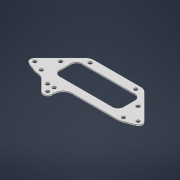
# Autodesk Inventor part: gusset-2-3.25-fulll-brace
Saved by Autodesk Inventor 2021 (Build 250183000, 183)
## iProperties
Created: 2020-11-04
Part Number: gusset-2-3.25-fulll-brace
Material: Generic
Document SubType Name: Modeling
Designer: Carlos Stewart
Density: 1 g/cm^3
Appearance: Default
Author: Carlos Stewart
Autodesk Inventor part; units mm, degrees
ref_plane "YZ Plane" through (0, 0, 0) normal (1, 0, 0) x (0, 1, 0)
ref_plane "XZ Plane" through (0, 0, 0) normal (0, 1, 0) x (-1, 0, 0)
ref_plane "XY Plane" through (0, 0, 0) normal (0, 0, 1) x (1, 0, 0)
sketch "Sketch1" plane through (0, 0, 0) normal (0, 1, 0) x (-1, 0, 0)
  line L0 (-37.8542, 0.1524) -> (35.8058, 0.1524)
  line L1 (43.4258, -7.4676) -> (43.4258, -23.2918)
  line L2 (35.8058, -30.9118) -> (-37.8542, -30.9118)
  line L3 (-45.4742, -23.2918) -> (-45.4742, -7.4676)
  arc A0 (-37.8542, 0.1524) -> (-45.4742, -7.4676) centre (-37.8542, -7.4676) ccw
  arc A1 (-45.4742, -23.2918) -> (-37.8542, -30.9118) centre (-37.8542, -23.2918) ccw
  arc A2 (35.8058, -30.9118) -> (43.4258, -23.2918) centre (35.8058, -23.2918) ccw
  arc A3 (43.4258, -7.4676) -> (35.8058, 0.1524) centre (35.8058, -7.4676) ccw
  circle A4 centre (-72.8662, -0.3634) radius 2.3114
  circle A5 centre (-54.9057, -18.324) radius 2.3114
  circle A6 centre (-58.1742, 5.2324) radius 2.3114
  circle A7 centre (56.1258, 5.2324) radius 2.3114
  circle A8 centre (-32.7742, -37.2618) radius 2.3114
  circle A9 centre (30.7258, -37.2618) radius 2.3114
  circle A10 centre (52.8574, -18.324) radius 2.3114
  circle A11 centre (70.8179, -0.3634) radius 2.3114
  circle A12 centre (34.8968, 17.5971) radius 2.3114
  circle A13 centre (25.9166, 26.5773) radius 2.3114
  circle A14 centre (25.9166, 17.5971) radius 2.3114
  arc A15 (75.308, -4.8536) -> (73.078, 5.5707) centre (70.8179, -0.3634) ccw
  arc A16 (58.386, 11.1665) -> (56.1258, 11.5824) centre (56.1258, 5.2324) ccw
  arc A17 (30.4067, 31.0675) -> (19.5666, 26.5773) centre (25.9166, 26.5773) ccw
  arc A18 (30.7258, -43.6118) -> (30.9592, -43.6075) centre (30.7258, -37.2618) ccw
  arc A19 (-75.1264, 5.5707) -> (-77.3564, -4.8536) centre (-72.8662, -0.3634) ccw
  arc A20 (-32.7742, -43.6118) -> (-31.4271, -43.4673) centre (-32.7742, -37.2618) ccw
  arc A21 (-58.1742, 11.5824) -> (-60.4344, 11.1665) centre (-58.1742, 5.2324) ccw
  line L4 (-75.1264, 5.5707) -> (-60.4344, 11.1665)
  line L5 (-77.3564, -4.8536) -> (-42.3179, -39.8921)
  line L6 (-33.3376, -43.6118) -> (31.2893, -43.6118)
  line L7 (75.308, -4.8536) -> (40.2695, -39.8921)
  line L8 (58.386, 11.1665) -> (73.078, 5.5707)
  line L9 (19.5666, 26.5773) -> (19.5666, 24.2824)
  line L10 (30.4067, 31.0675) -> (46.172, 15.3021)
  line L11 (55.1523, 11.5824) -> (56.1258, 11.5824)
  line L12 (-58.1742, 11.5824) -> (6.8666, 11.5824)
  arc A22 (-42.3179, -39.8921) -> (-33.3376, -43.6118) centre (-33.3376, -30.9118) ccw
  arc A23 (31.2893, -43.6118) -> (40.2695, -39.8921) centre (31.2893, -30.9118) ccw
  arc A24 (46.172, 15.3021) -> (55.1523, 11.5824) centre (55.1523, 24.2824) ccw
  arc A25 (6.8666, 11.5824) -> (19.5666, 24.2824) centre (6.8666, 24.2824) ccw
  point P0 (0, 0)
  point P1 (43.4258, -30.9118)
  point P2 (43.4258, 0.1524)
  point P3 (-45.4742, -30.9118)
  point P4 (43.4258, -30.9118)
  dimension "d2" = 7.62
  dimension "d20" = 12.7
  constraints: 32 point on circle, 30 tangent, 26 centre point, 26 end point, 8 coincident, 8 point on line, 6 equal radius, 4 perpendicular, 2 parallel, 1 horizontal, 1 vertical, 18 other
  measures "d2" radius of A0
  measures "d20" radius of A22
extrude "Extrusion1" add sketch "Sketch1" along normal blind 1.5875
body "Solid1"
